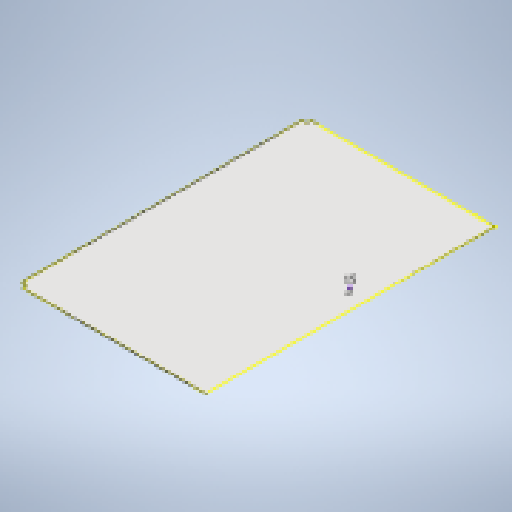
# Autodesk Inventor part: GnG frame 2 floor sheet 9
Saved by Autodesk Inventor 2025.3 (Build 293356030, 356C)
## iProperties
Created: 2025-10-28
Part Number: GnG frame 2 floor sheet 9
Material: Stainless Steel
Document SubType Name: Sheet Metal
Designer: admin
Mass: 280.619 g
Surface Area: 364.406 cm^2
Volume: 35.0774 cm^3
Density: 8 g/cm^3
Sheet Metal Rule: AISI304 3mm Die 32
Sheet Metal Width: 1500,000 mm
Sheet Metal Length: 2300,000 mm
Sheet Metal Area: 3450000,000 mm^2
Appearance: Default
Flat Pattern Width: 150 cm
Flat Pattern Length: 230 cm
Flat Pattern Area: 34500 cm^2
Author: admin
Autodesk Inventor part; units mm, degrees
ref_plane "YZ Plane" through (0, 0, 0) normal (1, 0, 0) x (0, 1, 0)
ref_plane "XZ Plane" through (0, 0, 0) normal (0, 1, 0) x (-1, 0, 0)
ref_plane "XY Plane" through (0, 0, 0) normal (0, 0, 1) x (1, 0, 0)
sketch "Sketch1" plane through (0, 0, 0) normal (0, 0, 1) x (1, 0, 0)
  line L0 (0, 0) -> (-1500, 0)
  line L1 (-1500, 0) -> (-1500, -2300)
  line L2 (-1500, -2300) -> (0, -2300)
  line L3 (0, -2300) -> (0, 0)
  line L4 (0, 0) -> (-40, 0)
  line L5 (-40, 0) -> (-40, -35)
  line L6 (-40, -35) -> (0, -35)
  line L7 (0, -35) -> (0, 0)
  line L8 (0, -2300) -> (-40, -2300)
  line L9 (-40, -2300) -> (-40, -2265)
  line L10 (-40, -2265) -> (0, -2265)
  line L11 (0, -2265) -> (0, -2300)
  line L12 (-1500, 0) -> (-1460, 0)
  line L13 (-1460, 0) -> (-1460, -35)
  line L14 (-1460, -35) -> (-1500, -35)
  line L15 (-1500, -35) -> (-1500, 0)
  line L16 (-1500, -2300) -> (-1460, -2300)
  line L17 (-1460, -2300) -> (-1460, -2265)
  line L18 (-1460, -2265) -> (-1500, -2265)
  line L19 (-1500, -2265) -> (-1500, -2300)
  line L20 (-550, -2300) -> (-450, -2300)
  line L21 (-450, -2300) -> (-450, -2265)
  line L22 (-450, -2265) -> (-550, -2265)
  line L23 (-550, -2265) -> (-550, -2300)
  line L24 (-550, 0) -> (-450, 0)
  line L25 (-450, 0) -> (-450, -35)
  line L26 (-450, -35) -> (-550, -35)
  line L27 (-550, -35) -> (-550, 0)
  point P0 (0, -35)
  point P1 (-40, 0)
  point P2 (-40, -2300)
  point P3 (0, -2265)
  point P4 (-450, -2300)
  point P5 (-450, 0)
  point P6 (-1460, 0)
  point P7 (-1500, -35)
  dimension "d22" = 1500
  dimension "d23" = 2300
  dimension "d24" = 40
  dimension "d25" = 35
  dimension "d28" = 100
  dimension "d29" = 410
  measures "d22" distance of L2.end L1.end
  measures "d23" distance of L1.end L0.end
  measures "d24" distance of L6.end L5.end
  measures "d25" distance of L5.end L4.end
  measures "d28" distance of L25.end L26.end
  measures "d29" distance between parallel lines of L5 L25
extrude "Plate1" add sketch "Sketch1" along normal blind 3 contours L3 L6 L5 L0 | L5 L6 L3 L10 L9 L2 L21 L22 L23 L17 L18 L1 L14 L13 L0 L27 L26 L25 | L25 L26 L27 L0 | L3 L2 L9 L10 | L2 L23 L22 L21
sketch "Sketch5" plane through (0, 0, 3) normal (0, 0, 1) x (1, 0, 0)
  line L0 (0, 0) -> (-100, 0) construction
  line L1 (-100, 0) -> (-100, -5) construction
  line L2 (-100, -5) -> (0, -5) construction
  line L3 (0, -5) -> (0, 0) construction
  line L4 (-100, 0) -> (-101.3084, -4.1277)
  arc A0 (-103.6916, -4.1277) -> (-101.3084, -4.1277) centre (-102.5, -3.75) ccw
  line L5 (-103.6916, -4.1277) -> (-105, 0)
  line L6 (-105, 0) -> (-100, 0)
  line L7 (-105, 0) -> (-110, 0) construction
  line L8 (-110, 0) -> (-115, 0)
  line L9 (-115, 0) -> (-115, -5)
  line L10 (-115, -5) -> (-110, -5)
  line L11 (-110, -5) -> (-110, 0)
  line L12 (-115, 0) -> (-120, 0) construction
  line L13 (-120, 0) -> (-125, 0)
  line L14 (-125, 0) -> (-125, -5)
  line L15 (-125, -5) -> (-120, -5)
  line L16 (-120, -5) -> (-120, 0)
  line L17 (-125, 0) -> (-130, 0) construction
  line L18 (-130, 0) -> (-135, 0)
  line L19 (-135, 0) -> (-135, -5)
  line L20 (-135, -5) -> (-130, -5)
  line L21 (-130, -5) -> (-130, 0)
  line L22 (-135, 0) -> (-140, 0) construction
  line L23 (-140, 0) -> (-145, 0)
  line L24 (-145, 0) -> (-145, -5)
  line L25 (-145, -5) -> (-140, -5)
  line L26 (-140, -5) -> (-140, 0)
  line L27 (-145, 0) -> (-150, 0) construction
  line L28 (-150, 0) -> (-155, 0) construction
  circle A1 centre (-150, 0) radius 2.5
  point P0 (-102.5, 0)
  dimension "d30" = 100
  dimension "d31" = 5
  dimension "d32" = 5
  dimension "d33" = 5
  dimension "d34" = 1.25
  dimension "d35" = 5
  dimension "d36" = 5
  dimension "d37" = 5
  dimension "d38" = 5
  constraints: 58 end point, 11 horizontal, 10 equal length, 10 parallel, 5 perpendicular, 3 coincident, 3 tangent, 2 centre point, 2 point on circle, 1 midpoint, 1 point on line, 1 vertical alignment
  measures "d30" distance of L2.end L1.end
  measures "d31" distance of L1.end L0.end
  measures "d32" distance of L9.end L9.start
  measures "d33" distance of L5.end L0.end
  measures "d34" radius of A0
  measures "d35" distance of L15.start L13.end
  measures "d36" distance of L19.end L19.start
  measures "d37" distance of L24.end L24.start
  measures "d38" diameter of A1
extrude "Cut1" cut sketch "Sketch5" against normal blind 3 contours L4 A0 L5 L6 | L11 L10 L9 L8 | A1
sketch "Sketch6" plane through (0, 0, 3) normal (0, 0, 1) x (1, 0, 0)
  arc A0 (-152.5, 0) -> (-147.5, 0) centre (-150, 0) ccw projected
  line L0 (-1460, 0) -> (-152.5, 0) projected
  line L1 (-1460, -35) -> (-1460, 0) projected
  line L2 (-1500, -35) -> (-1460, -35) projected
  line L3 (-1500, -2265) -> (-1500, -35) projected
  line L4 (-1460, -2265) -> (-1500, -2265) projected
  line L5 (-1460, -2300) -> (-1460, -2265) projected
  line L6 (0, -2300) -> (-1460, -2300) projected
  line L7 (0, 0) -> (0, -2300) projected
  line L8 (-100, 0) -> (0, 0) projected
  line L9 (-100, 0) -> (-101.3084, -4.1277) projected
  arc A1 (-103.6916, -4.1277) -> (-101.3084, -4.1277) centre (-102.5, -3.75) ccw projected
  line L10 (-103.6916, -4.1277) -> (-105, 0) projected
  line L11 (-110, 0) -> (-105, 0) projected
  line L12 (-110, 0) -> (-110, -5) projected
  line L13 (-110, -5) -> (-115, -5) projected
  line L14 (-115, -5) -> (-115, 0) projected
  line L15 (-147.5, 0) -> (-115, 0) projected
  circle A2 centre (-630, -1000) radius 7.5
  dimension "d41" = 15
  dimension "d42" = 1000
  dimension "d43" = 630
  constraints: 1 centre point
  measures "d41" diameter of A2
  measures "d42" distance from line of L0 A2.centre
  measures "d43" distance from line of A2.centre L7
extrude "Cut2" cut sketch "Sketch6" against normal blind 3 contours A2
equation "\"d34\" = 0.25 * d31"
equation "\"d39\" = Thickness"
equation "\"d44\" = Thickness"
equation "\"d2\" = Thickness"
equation "\"BendReliefWidth\" = Thickness"
equation "\"BendReliefDepth\" = 0.5 * Thickness"
equation "\"CornerReliefSize\" = 4 * Thickness"
equation "\"MinimumRemnant\" = 2 * Thickness"
equation "\"TransitionRadius\" = BendRadius"
equation "\"JacobiRadiusSize\" = BendRadius"
equation "\"GapSize\" = Thickness"
equation "\"Thickness\" = 3"
equation "\"BendRadius\" = 5"
body "Solid1"
